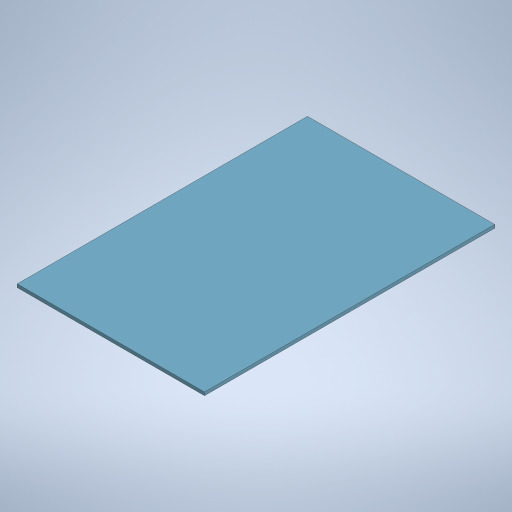
# Autodesk Inventor part: BaseCase
Saved by Autodesk Inventor 2024 (Build 280153000, 153)
## iProperties
Created: 2024-02-15
Part Number: BaseCase
Material: Generic
Document SubType Name: Modeling
Designer: fabiancastano
Density: 1 g/cm^3
Appearance: Default
Author: fabiancastano
Autodesk Inventor part; units mm, degrees
ref_plane "YZ Plane" through (0, 0, 0) normal (1, 0, 0) x (0, 1, 0)
ref_plane "XZ Plane" through (0, 0, 0) normal (0, 1, 0) x (-1, 0, 0)
ref_plane "XY Plane" through (0, 0, 0) normal (0, 0, 1) x (1, 0, 0)
sketch "Sketch1" plane through (0, 0, 0) normal (0, 1, 0) x (-1, 0, 0)
  line L0 (100, 155) -> (-100, 155)
  line L1 (-100, 155) -> (-100, -155)
  line L2 (-100, -155) -> (100, -155)
  line L3 (100, -155) -> (100, 155)
  point P0 (0, 0)
  point P1 (100, 0)
  point P2 (0, -155)
  dimension "d0" = 200
  dimension "d1" = 310
  constraints: 8 end point, 2 midpoint, 2 parallel, 1 horizontal, 1 horizontal alignment, 1 perpendicular, 1 vertical alignment
  measures "d0" distance of L2.end L1.end
  measures "d1" distance of L1.end L0.end
extrude "Extrusion1" add sketch "Sketch1" along normal blind 3.5
body "Solid1"
